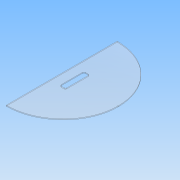
# Autodesk Inventor part: Top_Guard 3
Saved by Autodesk Inventor 2018.1 (Build 221171000, 171)
## iProperties
Created: 2019-03-23
Part Number: Top_Guard 3
Material: PMMA Plastic
Document SubType Name: Modeling
Designer: James
Density: 1.188 g/cm^3
Appearance: Polycarbonate - Clear
Author: James
Autodesk Inventor part; units mm, degrees
ref_plane "YZ Plane" through (0, 0, 0) normal (1, 0, 0) x (0, 1, 0)
ref_plane "XZ Plane" through (0, 0, 0) normal (0, 1, 0) x (-1, 0, 0)
ref_plane "XY Plane" through (0, 0, 0) normal (0, 0, 1) x (1, 0, 0)
sketch "Sketch1" plane through (0, 0, 0) normal (0, 0, 1) x (1, 0, 0)
  ellipse E0 centre (0, 0) end of major axis (612, 0) minor radius 600
  dimension "d0" = 612
  dimension "d1" = 600
  constraints: 1 coincident, 2 other
extrude "Extrusion1" add sketch "Sketch1" along normal blind 10
sketch "Sketch2" plane through (0, 0, 10) normal (0, 0, 1) x (1, 0, 0)
  line L0 (-612, 600) -> (0, 600)
  line L1 (0, 600) -> (0, -600)
  line L2 (0, -600) -> (-612, -600)
  line L3 (-612, -600) -> (-612, 600)
  ellipse E0 centre (0, 0) end of major axis (-612, 0) minor radius 600 projected
  constraints: 8 end point, 2 horizontal, 2 parallel, 1 coincident, 1 midpoint, 1 perpendicular, 1 vertical, 1 other
extrude "Extrusion2" cut sketch "Sketch2" against normal through all contours L0 E0 L3 | L1 E0 | E0 L2 L3 picked at (-19.6985, 199.8178)
sketch "Sketch3" plane through (0, 0, 10) normal (0, 0, 1) x (1, 0, 0)
  line L0 (105, -125) -> (165, -125)
  line L1 (165, -125) -> (165, 135)
  line L2 (165, 135) -> (105, 135)
  line L3 (105, 135) -> (105, -125)
  line L4 (0, 600) -> (0, -600) projected
  point P0 (0, 0)
  dimension "d8" = 105
  dimension "d9" = 60
  dimension "d10" = 260
  dimension "d11" = 125
  constraints: 8 end point, 2 parallel, 1 horizontal, 1 perpendicular
  measures "d8" distance between parallel lines of L4 L3
  measures "d9" distance of L0.start L0.end
  measures "d10" distance of L0.end L1.end
  measures "d11" distance from line of point (0, 0) L0
extrude "Extrusion3" cut sketch "Sketch3" against normal through all
fillet "Fillet1" radius 15 4 edges at (105, -125, 5) (165, -125, 5) (165, 135, 5) (105, 135, 5)
ref_plane "Work Plane1" through (612, -600, 10) normal (-1, 0, 0) x (0, 0, 1)
sketch "Sketch4" plane through (612, -600, 10) normal (-1, 0, 0) x (0, 0, 1)
  line L0 (0, 0) -> (0, 1200) projected
  line L1 (-12, 600) -> (2, 600) projected
  point P0 (-10, 600)
  point P1 (-5, 600)
  dimension "d16" = 5
  constraints: 1 midpoint
  measures "d16" distance from line of point (-5, 600) L0
hole "Hole1" at (612, 0, 5) direction (-1, 0, 0) diameter 3.242 depth 11.8 tip angle 118 thread size "M4x0.7" class "6H" standard "ANSI Metric M Profile"
body "Solid1"
